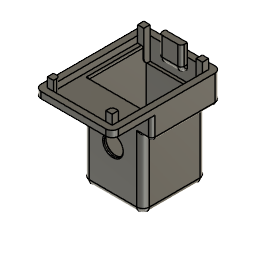
soilmeter_bottom (Autodesk Fusion 360 design; units mm, degrees)
part number: 2026-05-26-23-54-00-589
Autodesk Fusion 360 part; units mm, degrees
sketch "Sketch1" plane through (0, 0, 0) normal (0, 0, 1) x (1, 0, 0)
  line L0 (13.0835, 14.3647) -> (54.0835, 14.3647)
  line L1 (54.0835, 14.3647) -> (54.0835, -46.6353)
  line L2 (54.0835, -46.6353) -> (13.0835, -46.6353)
  line L3 (13.0835, -46.6353) -> (13.0835, 14.3647)
  line L4 (9.0835, 18.3647) -> (58.0835, 18.3647)
  line L5 (58.0835, 18.3647) -> (58.0835, -50.6353)
  line L6 (58.0835, -50.6353) -> (9.0835, -50.6353)
  line L7 (9.0835, -50.6353) -> (9.0835, 18.3647)
  line L8 (13.0835, -46.6353) -> (17.0835, -46.6353)
  line L9 (17.0835, -46.6353) -> (17.0835, -42.6353)
  line L10 (17.0835, -42.6353) -> (13.0835, -42.6353)
  line L11 (13.0835, -42.6353) -> (13.0835, -46.6353)
  line L12 (54.0835, -46.6353) -> (50.0835, -46.6353)
  line L13 (50.0835, -46.6353) -> (50.0835, -42.6353)
  line L14 (50.0835, -42.6353) -> (54.0835, -42.6353)
  line L15 (54.0835, -42.6353) -> (54.0835, -46.6353)
  line L16 (13.0835, 14.3647) -> (17.0835, 14.3647)
  line L17 (17.0835, 14.3647) -> (17.0835, 10.3647)
  line L18 (17.0835, 10.3647) -> (13.0835, 10.3647)
  line L19 (13.0835, 10.3647) -> (13.0835, 14.3647)
  line L20 (54.0835, 14.3647) -> (50.0835, 14.3647)
  line L21 (50.0835, 14.3647) -> (50.0835, 10.3647)
  line L22 (50.0835, 10.3647) -> (54.0835, 10.3647)
  line L23 (54.0835, 10.3647) -> (54.0835, 14.3647)
  line L24 (26.5835, 14.3647) -> (40.5835, 14.3647)
  line L25 (40.5835, 14.3647) -> (40.5835, 10.3647)
  line L26 (40.5835, 10.3647) -> (26.5835, 10.3647)
  line L27 (26.5835, 10.3647) -> (26.5835, 14.3647)
  line L28 (58.0835, -50.6353) -> (9.0835, -50.6353)
  line L29 (9.0835, -50.6353) -> (9.0835, -25.6353)
  line L30 (9.0835, -25.6353) -> (58.0835, -25.6353)
  line L31 (58.0835, -25.6353) -> (58.0835, -50.6353)
  line L32 (13.0835, -25.6353) -> (15.0835, -25.6353)
  line L33 (15.0835, -25.6353) -> (15.0835, 10.3647)
  line L34 (15.0835, 10.3647) -> (13.0835, 10.3647)
  line L35 (13.0835, 10.3647) -> (13.0835, -25.6353)
  line L36 (54.0835, 10.3647) -> (52.0835, 10.3647)
  line L37 (52.0835, 10.3647) -> (52.0835, -25.6353)
  line L38 (52.0835, -25.6353) -> (54.0835, -25.6353)
  line L39 (54.0835, -25.6353) -> (54.0835, 10.3647)
  line L40 (13.0835, 14.3647) -> (54.0835, 14.3647)
  line L41 (54.0835, 14.3647) -> (54.0835, 10.3647)
  line L42 (54.0835, 10.3647) -> (13.0835, 10.3647)
  line L43 (13.0835, 10.3647) -> (13.0835, 14.3647)
  dimension "d1" = 41
  dimension "d2" = 61
  dimension "d3" = 4
  dimension "d5" = 4
  dimension "d6" = 4
  dimension "d7" = 4
  dimension "d8" = 4
  dimension "d9" = 4
  dimension "d10" = 4
  dimension "d11" = 4
  dimension "d12" = 4
  dimension "d13" = 4
  dimension "d14" = 4
  dimension "d15" = 4
  dimension "d16" = 14
  dimension "d17" = 4
  dimension "d18" = 9.5
  dimension "d25" = 49
  dimension "d26" = 25
  dimension "d27" = 2
  dimension "d28" = 36
  dimension "d29" = 2
  dimension "d30" = 36
  constraint horizontal L0
  constraint vertical L1
  constraint horizontal L2
  constraint vertical L3
  constraint horizontal L4
  constraint vertical L5
  constraint horizontal L6
  constraint vertical L7
  constraint horizontal L8
  constraint vertical L9
  constraint horizontal L10
  constraint vertical L11
  constraint horizontal L12
  constraint vertical L13
  constraint horizontal L14
  constraint vertical L15
  constraint horizontal L16
  constraint vertical L17
  constraint horizontal L18
  constraint vertical L19
  constraint horizontal L20
  constraint vertical L21
  constraint horizontal L22
  constraint vertical L23
  constraint horizontal L24
  constraint vertical L25
  constraint horizontal L26
  constraint vertical L27
  constraint coincident L0 L24.start
  constraint horizontal L28
  constraint vertical L29
  constraint horizontal L30
  constraint vertical L31
  constraint horizontal L32
  constraint vertical L33
  constraint horizontal L34
  constraint vertical L35
  constraint coincident L30 L32.start
  constraint coincident L3 L32.start
  constraint horizontal L36
  constraint vertical L37
  constraint horizontal L38
  constraint vertical L39
  constraint horizontal L40
  constraint vertical L41
  constraint horizontal L42
  constraint vertical L43
  measures "d1" distance of L0.start L0.end
  measures "d2" distance of L0.start L2.end
  measures "d3" distance of L2 L6
  measures "d5" distance of L3 L7
  measures "d6" distance of L1 L5
  measures "d7" distance of L0 L4
  measures "d8" distance of L2.end L8.end
  measures "d9" distance of L2.end L10.end
  measures "d10" distance of L1.end L12.end
  measures "d11" distance of L1.end L14.end
  measures "d12" distance of L0.start L16.end
  measures "d13" distance of L0.start L18.end
  measures "d14" distance of L0.end L20.end
  measures "d15" distance of L0.end L22.end
  measures "d16" distance of L24.start L24.end
  measures "d17" distance of L24.start L26.end
  measures "d18" distance of L17 L27
  measures "d25" distance of L5.end L6.end
  measures "d26" distance of L5.end L30.end
  measures "d27" distance of L32.start L32.end
  measures "d28" distance of L32.start L18.end
  measures "d29" distance of L22.end L36.end
  measures "d30" distance of L22.end L38.end
extrude "Extrude1" add sketch "Sketch1" along normal blind 4 contours L0 L1 L3 L4 L5 L7 L16 L19 L20 L23 L24 L30 L35 L39 L40 L41 L43 | L1 L2 L3 L5 L6 L7 L8 L11 L12 L15 L28 L29 L30 L31 makes body 1
extrude "Extrude2" add sketch "Sketch1" along normal blind 10 separate body contours L0 L3 L16 L17 L18 L19 L34 L40 L42 L43 | L2 L3 L8 L9 L10 L11 | L0 L1 L20 L21 L22 L23 L36 L40 L41 L42 | L1 L2 L12 L13 L14 L15 makes body 2 at (51.4168, 14.3647, 3.3333) makes body 3 at (50.0835, -45.3019, 3.3333) makes body 4 at (14.4168, 14.3647, 3.3333) makes body 5 at (17.0835, -45.3019, 3.3333)
extrude "Extrude3" add sketch "Sketch1" along normal blind 12 contours L0 L24 L25 L26 L27 L40 L42 bodies 1
extrude "Extrude4" add sketch "Sketch1" against normal blind 10 contours L0 L1 L3 L4 L5 L7 L16 L19 L20 L23 L24 L30 L35 L39 L40 L41 L43 | L0 L3 L16 L17 L18 L19 L34 L40 L42 L43 | L3 L18 L30 L32 L33 L34 L35 L42 | L0 L1 L20 L21 L22 L23 L36 L40 L41 L42 | L1 L22 L30 L36 L37 L38 L39 L42 bodies 1 2 4
sketch "Sketch2" plane through (0, 0, -10) normal (0, 0, -1) x (1, 0, 0)
  line L0 (50.0835, -14.3647) -> (17.0835, -14.3647)
  line L1 (17.0835, -14.3647) -> (17.0835, -10.3647)
  line L2 (17.0835, -10.3647) -> (15.0835, -10.3647)
  line L3 (15.0835, -10.3647) -> (15.0835, 25.6353)
  line L4 (15.0835, 25.6353) -> (9.0835, 25.6353)
  line L5 (9.0835, 25.6353) -> (9.0835, -18.3647)
  line L6 (9.0835, -18.3647) -> (58.0835, -18.3647)
  line L7 (58.0835, -18.3647) -> (58.0835, 25.6353)
  line L8 (58.0835, 25.6353) -> (52.0835, 25.6353)
  line L9 (52.0835, 25.6353) -> (52.0835, -10.3647)
  line L10 (52.0835, -10.3647) -> (50.0835, -10.3647)
  line L11 (50.0835, -10.3647) -> (50.0835, -14.3647)
  line L12 (9.0835, -18.3647) -> (58.0835, -18.3647)
  line L13 (16.5835, 25.6353) -> (50.5835, 25.6353)
  line L14 (50.5835, 25.6353) -> (50.5835, -12.3647)
  line L15 (50.5835, -12.3647) -> (16.5835, -12.3647)
  line L16 (16.5835, -12.3647) -> (16.5835, 25.6353)
  line L17 (9.0835, 50.6353) -> (9.0835, -18.3647)
  line L18 (9.0835, 25.6353) -> (58.0835, 25.6353)
  line L19 (58.0835, 25.6353) -> (58.0835, 23.6353)
  line L20 (58.0835, 23.6353) -> (9.0835, 23.6353)
  line L21 (9.0835, 23.6353) -> (9.0835, 25.6353)
  dimension "d41" = 34
  dimension "d42" = 7.5
  dimension "d43" = 49
  dimension "d44" = 2
  constraint horizontal L13
  constraint vertical L14
  constraint horizontal L15
  constraint vertical L16
  constraint horizontal L18
  constraint vertical L19
  constraint horizontal L20
  constraint vertical L21
  constraint coincident L4.end L5.start
  measures "d41" distance of L13.start L13.end
  measures "d42" distance of L16 L17
  measures "d43" distance of L4.end L7.end
  measures "d44" distance of L4.end L20.end
extrude "Extrude5" add sketch "Sketch2" along normal blind 4 contours L0 L1 L2 L3 L5 L6 L7 L9 L10 L11 L12 L14 L15 L16 L17 L20 | L0 L1 L11 L15 | L9 L10 L14 L20 | L2 L3 L16 L20 | L13 L14 L16 L18 L20 | L9 L14 L18 L20 | L3 L16 L18 L20 | L7 L8 L9 L18 L19 L20 | L3 L4 L5 L17 L18 L20 L21 bodies 1
sketch "Sketch3" plane through (0, 0, -14) normal (0, 0, -1) x (1, 0, 0)
  line L0 (16.5835, 23.6353) -> (50.5835, 23.6353)
  line L1 (50.5835, 23.6353) -> (50.5835, -12.3647)
  line L2 (50.5835, -12.3647) -> (16.5835, -12.3647)
  line L3 (16.5835, -12.3647) -> (16.5835, 23.6353)
  line L4 (9.0835, -18.3647) -> (58.0835, -18.3647)
  line L5 (58.0835, -18.3647) -> (58.0835, 25.6353)
  line L6 (58.0835, 25.6353) -> (9.0835, 25.6353)
  line L7 (9.0835, 25.6353) -> (9.0835, -18.3647)
  line L8 (14.5835, -14.3647) -> (52.5835, -14.3647)
  line L9 (52.5835, -14.3647) -> (52.5835, 25.6353)
  line L10 (52.5835, 25.6353) -> (14.5835, 25.6353)
  line L11 (14.5835, 25.6353) -> (14.5835, -14.3647)
  line L12 (9.0835, 50.6353) -> (9.0835, -18.3647)
  line L13 (58.0835, -18.3647) -> (58.0835, 50.6353)
  line L14 (52.5835, -14.3647) -> (14.5835, -14.3647)
  line L15 (14.5835, -14.3647) -> (14.5835, -12.3647)
  line L16 (14.5835, -12.3647) -> (52.5835, -12.3647)
  line L17 (52.5835, -12.3647) -> (52.5835, -14.3647)
  dimension "d47" = 5.5
  dimension "d48" = 5.5
  dimension "d49" = 2
  constraint horizontal L8
  constraint vertical L9
  constraint horizontal L10
  constraint vertical L11
  constraint coincident L6 L9.end
  constraint horizontal L14
  constraint vertical L15
  constraint horizontal L16
  constraint vertical L17
  constraint coincident L11 L15.end
  measures "d47" distance of L11 L12
  measures "d48" distance of L9 L13
  measures "d49" distance of L2 L8
extrude "Extrude6" add sketch "Sketch3" along normal blind 40 contours L0 L1 L3 L6 L9 L10 L11 L16 | L2 L8 L9 L11 L14 L15 L16 L17 bodies 1
sketch "Sketch4" plane through (0, 0, -54) normal (0, 0, -1) x (1, 0, 0)
  line L0 (50.5835, -12.3647) -> (16.5835, -12.3647)
  line L1 (16.5835, -12.3647) -> (16.5835, 23.6353)
  line L2 (16.5835, 23.6353) -> (50.5835, 23.6353)
  line L3 (50.5835, 23.6353) -> (50.5835, -12.3647)
  line L4 (14.5835, 25.6353) -> (14.5835, -14.3647)
  line L5 (14.5835, -14.3647) -> (52.5835, -14.3647)
  line L6 (52.5835, -14.3647) -> (52.5835, 25.6353)
  line L7 (52.5835, 25.6353) -> (14.5835, 25.6353)
extrude "Extrude7" add sketch "Sketch4" along normal blind 4 contours L0 L1 L2 L3 | L4 L5 L6 L7 bodies 1
fillet "Fillet1" radius 4 4 edges at (33.5835, 14.3647, -58) (52.5835, -5.6353, -58) (33.5835, -25.6353, -58) (14.5835, -5.6353, -58) on bodies 1
extrude "Extrude8" add 1 faces at (27.9168, -24.9686, -10) along direction (0, 0, 1) blind 10 on bodies 1 bodies 1
extrude "Extrude9" add sketch "Sketch1" against normal blind 4 contours L1 L2 L3 L9 L10 L13 L14 L30 L32 L38 | L2 L3 L8 L9 L10 L11 | L1 L2 L12 L13 L14 L15 bodies 1 3 5
sketch "Sketch5" plane through (0, -25.6353, 0) normal (0, -1, 0) x (1, 0, 0)
  line L0 (13.0835, -4) -> (13.0835, 0)
  line L1 (13.0835, 0) -> (9.0835, 0)
  line L2 (9.0835, 0) -> (9.0835, -14)
  line L3 (9.0835, -14) -> (14.5835, -14)
  line L4 (14.5835, -14) -> (14.5835, -54)
  line L5 (14.5835, -54) -> (52.5835, -54)
  line L6 (52.5835, -54) -> (52.5835, -14)
  line L7 (52.5835, -14) -> (58.0835, -14)
  line L8 (58.0835, -14) -> (58.0835, 0)
  line L9 (58.0835, 0) -> (54.0835, 0)
  line L10 (54.0835, 0) -> (54.0835, -4)
  line L11 (54.0835, -4) -> (13.0835, -4)
  circle A0 centre (33.5835, -28) radius 6
  line L12 (16.5835, -54) -> (16.5835, 0)
  dimension "d60" = 12
  dimension "d61" = 17
  dimension "d62" = 24
  measures "d60" diameter of A0
  measures "d61" distance of A0.centre L12
  measures "d62" distance of L11 A0.centre
extrude "Extrude10" cut sketch "Sketch5" against normal blind 12 contours A0 bodies 1
fillet "Fillet2" radius 0.5 2 edges at (27.9895, -25.6353, -25.8303) (27.9895, -23.6353, -30.1697) on bodies 1
fillet "Fillet3" radius 4 2 edges at (58.0835, -50.6353, 2) (9.0835, -50.6353, 2) on bodies 1
fillet "Fillet4" radius 4 2 edges at (58.0835, 18.3647, -5) (9.0835, 18.3647, -5) on bodies 1
fillet "Fillet5" radius 4 8 edges at (14.5835, -25.6353, -34) (15.7551, -24.4637, -56.8284) (51.4119, -24.4637, -56.8284) (52.5835, -25.6353, -34) (52.5835, 14.3647, -34) (51.4119, 13.1932, -56.8284) (14.5835, 14.3647, -34) (15.7551, 13.1932, -56.8284) on bodies 1
fillet "Fillet6" radius 2 1 edges at (9.0835, -25.6353, -7) on bodies 1
fillet "Fillet7" radius 2 1 edges at (58.0835, -25.6353, -7) on bodies 1
fillet "Fillet8" radius 4 2 edges at (13.0835, -46.6353, -2) (54.0835, -46.6353, -2) on bodies 1
fillet "Fillet9" radius 2 9 edges at (14.8335, -25.6353, -14) (9.6693, -25.0495, -14) (9.0835, -4.6353, -14) (10.2551, 17.1932, -14) (33.5835, 18.3647, -14) (56.9119, 17.1932, -14) (58.0835, -4.6353, -14) (57.4977, -25.0495, -14) (52.3335, -25.6353, -14) on bodies 1
extrude "Extrude11" add sketch "Sketch1" against normal blind 4 separate body contours L0 L24 L25 L26 L27 L40 L42 makes body 6
fillet "Fillet10" radius 4 1 edges at (33.5835, 10.3647, -4) on bodies 6
fillet "Fillet11" radius 2 1 edges at (17.0835, -42.6353, 5) on bodies 1
fillet "Fillet12" radius 2 1 edges at (50.0835, -42.6353, 5) on bodies 1
fillet "Fillet13" radius 4 1 edges at (16.8335, 10.3647, -10) on bodies 1
fillet "Fillet14" radius 4 1 edges at (50.3335, 10.3647, -10) on bodies 1
fillet "Fillet15" radius 2 2 edges at (26.5835, 10.3647, 6) (26.5835, 11.5363, -2.8284) on bodies 1 6
fillet "Fillet16" radius 2 2 edges at (40.5835, 10.3647, 6) (40.5835, 11.5363, -2.8284) on bodies 1 6
fillet "Fillet17" radius 1 3 edges at (16.5835, -6.6353, 0) (33.5835, -23.6353, 0) (50.5835, -6.6353, 0) on bodies 1
fillet "Fillet18" radius 1 5 edges at (54.0835, -34.1353, -4) (52.9119, -45.4637, -4) (33.5835, -46.6353, -4) (14.2551, -45.4637, -4) (13.0835, -34.1353, -4) on bodies 1
